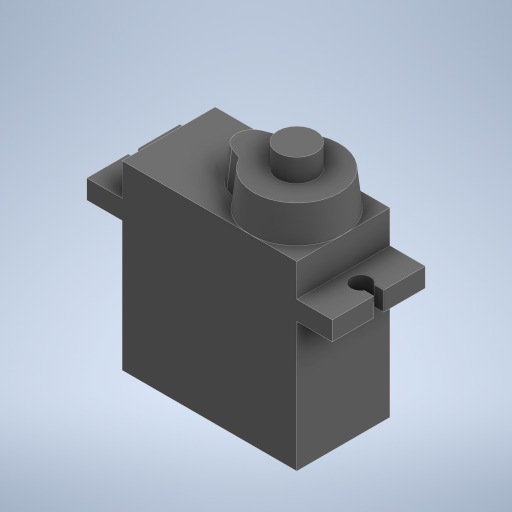
# Autodesk Inventor part: Servo_small_maketa
Saved by Autodesk Inventor 2023 (Build 270158000, 158)
## iProperties
Created: 2024-06-26
Part Number: Servo_small_maketa
Material: Generic
Document SubType Name: Modeling
Designer: Swoby
Density: 1 g/cm^3
Appearance: Default
Author: Swoby
Autodesk Inventor part; units mm, degrees
ref_plane "YZ Plane" through (0, 0, 0) normal (1, 0, 0) x (0, 1, 0)
ref_plane "XZ Plane" through (0, 0, 0) normal (0, 1, 0) x (-1, 0, 0)
sketch "Sketch1" plane through (0, 0, 0) normal (0, 1, 0) x (-1, 0, 0)
  line L0 (-11.45, 6.1) -> (11.45, 6.1)
  line L1 (11.45, 6.1) -> (11.45, -6.1)
  line L2 (11.45, -6.1) -> (-11.45, -6.1)
  line L3 (-11.45, -6.1) -> (-11.45, 6.1)
  line L4 (-11.45, 6.1) -> (11.45, -6.1) construction
  line L5 (11.45, 6.1) -> (-11.45, -6.1) construction
  point P0 (0, 0)
  dimension "d0" = 22.9
  dimension "d1" = 12.2
  constraints: 12 end point, 2 midpoint, 2 parallel, 1 horizontal, 1 perpendicular
  measures "d0" distance of L1.end L2.end
  measures "d1" distance of L0.end L1.end
extrude "Extrusion1" add sketch "Sketch1" along normal blind 28.3
ref_plane "Work Plane1" through (0, 17, 0) normal (0, -1, 0) x (1, 0, 0)
sketch "Sketch2" plane through (0, 17, 0) normal (0, -1, 0) x (1, 0, 0)
  line L0 (-11.45, 6.1) -> (11.45, 6.1) projected
  line L1 (11.45, 6.1) -> (16.1, 6.1)
  line L2 (16.1, 6.1) -> (16.1, -6.1)
  line L3 (16.1, -6.1) -> (11.45, -6.1)
  line L4 (11.45, -6.1) -> (11.45, 6.1)
  line L5 (-11.45, -6.1) -> (-11.45, 6.1) projected
  line L6 (-11.45, 6.1) -> (-16.1, 6.1)
  line L7 (-16.1, 6.1) -> (-16.1, 0.65)
  line L8 (-16.1, -6.1) -> (-11.45, -6.1)
  line L9 (-11.45, -6.1) -> (-11.45, 6.1)
  line L10 (11.45, -6.1) -> (-11.45, -6.1) projected
  arc A0 (-15.05, 0) -> (-14.8758, -0.65) centre (-13.75, 0) ccw construction
  line L11 (-16.1, -0.65) -> (-14.8758, -0.65)
  line L12 (-16.1, 0.65) -> (-14.8758, 0.65)
  line L13 (-16.1, 0) -> (16.1, 0) construction
  line L14 (-16.1, -0.65) -> (-16.1, -6.1)
  line L15 (-16.1, 0.65) -> (-16.1, -0.65) construction
  arc A1 (-14.8758, 0.65) -> (-15.05, 0) centre (-13.75, 0) ccw construction
  arc A2 (-14.8758, -0.65) -> (-14.8758, 0.65) centre (-13.75, 0) ccw
  circle A3 centre (13.75, 0) radius 1.3
  line L16 (14.8758, -0.65) -> (16.1, -0.65)
  line L17 (14.8758, 0.65) -> (16.1, 0.65)
  point P0 (0, 0)
  point P1 (-11.45, 0)
  point P2 (-15.4879, -0.65)
  dimension "d5" = 32.2
  dimension "d6" = 22.9
  dimension "d7" = 4.65
  dimension "d14" = 2.6
  dimension "d15" = 2.3
  dimension "d16" = 1.3
  dimension "d17" = 0.65
  dimension "d18" = 2.6
  dimension "d19" = 2.3
  dimension "d20" = 1.3
  dimension "d21" = 0.65
  constraints: 30 end point, 8 point on circle, 7 parallel, 6 perpendicular, 6 point on line, 4 centre point, 3 horizontal, 3 midpoint
  measures "d5" distance between parallel lines of L7 L2
  measures "d6" distance of L3.end L5.start
  measures "d7" distance of L2.end L3.end
  measures "d14" diameter of A0
  measures "d15" distance of point (-11.45, 0) A0.centre
  measures "d16" distance from line of L12 point (-15.488, -0.65)
  measures "d17" distance from line of L11 A0.centre
  measures "d18" diameter of A3
  measures "d19" distance from line of L4 A3.centre
  measures "d20" distance between parallel lines of L17 L16
  measures "d21" distance between parallel lines of L16 L13
extrude "Extrusion2" add sketch "Sketch2" against normal blind 2.5 contours L5 L8 L14 L11 A2 L12 L7 L6 | L1 L2 L17 A3 L16 L3 L4
sketch "Sketch3" plane through (0, 28.3, 0) normal (0, 1, 0) x (1, 0, 0)
  circle A0 centre (5.35, 0) radius 2.5
  line L0 (16.1, -6.1) -> (16.1, 6.1) projected
  line L1 (-11.45, 6.1) -> (-11.45, -6.1) construction
  line L2 (-11.45, 0) -> (16.1, 0)
  circle A1 centre (5.35, 0) radius 6.1 construction
  line L3 (11.45, 6.1) -> (-11.45, 6.1) construction
  line L4 (-11.45, -6.1) -> (11.45, -6.1) construction
  line L5 (11.45, -6.1) -> (11.45, 6.1) construction
  point P0 (0, 0)
  dimension "d10" = 5
  constraints: 2 centre point, 2 end point, 2 midpoint, 2 tangent, 1 point on line
  measures "d10" diameter of A0
extrude "Extrusion3" add sketch "Sketch3" along normal blind 3
sketch "Sketch4" plane through (0, 28.3, 0) normal (0, 1, 0) x (1, 0, 0)
  circle A0 centre (5.35, 0) radius 2.5 projected
  circle A1 centre (5.35, 0) radius 6.1
  circle A2 centre (-0.4, 0) radius 2.65
  line L0 (11.45, 6.1) -> (-11.45, 6.1) projected
  line L1 (-0.4, 0) -> (5.35, 0)
  line L2 (-0.4, 0) -> (-3.05, 0)
  line L3 (5.35, 0) -> (11.45, 0)
  line L4 (-1.3388, 2.4781) -> (0.0387, 3)
  line L5 (-1.3388, -2.4781) -> (0.0387, -3)
  line L6 (11.45, 6.1) -> (-11.45, 6.1) projected
  line L7 (11.45, -6.1) -> (11.45, 6.1) projected
  line L8 (-11.45, -6.1) -> (11.45, -6.1) projected
  line L9 (-11.45, 6.1) -> (-11.45, -6.1) projected
  point P0 (0, 0)
  point P1 (5.35, -6.1)
  point P2 (5.35, 6.1)
  dimension "d22" = 14.5
  dimension "d23" = 5.3
  dimension "d24" = 6
  dimension "d25" = 3
  constraints: 10 end point, 6 point on circle, 3 horizontal, 3 tangent, 2 centre point, 1 coincident
  measures "d22" distance of L3.end L2.end
  measures "d23" diameter of A2
  measures "d24" distance of L5.end L4.end
  measures "d25" vertical distance of L4.end point (0, 0)
extrude "Extrusion4" cut sketch "Sketch4" against normal blind 4.5 contours L7 L8 A1 | A1 L0 L7 | A1 L4 A2 L5 L8 L9 L0
chamfer "Chamfer1" distance 0.5 distance2 4.5 5 edges at (-0.6501, 28.3, 2.7391) (-3.05, 28.3, 0) (-0.6501, 28.3, -2.7391) (10.6183, 28.3, -3.0749) (2.2751, 28.3, 5.2683) measured on face at (0.0574, 28.3, 0)
equation "\"d7\" = -0.5 * d6 + 0.5 * d5"
equation "\"d17\" = 0.5 * d16"
equation "\"d21\" = 0.5 * d20"
body "Solid1"
